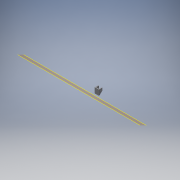
# Autodesk Inventor part: Y belt mount point
Saved by Autodesk Inventor 2016 (Build 200138000, 138)
## iProperties
Created: 2016-05-31
Part Number: Y belt mount point
Material: Generic
Document SubType Name: Modeling
Designer: Scott
Density: 1 g/cm^3
Appearance: Default
Author: Scott
Autodesk Inventor part; units mm, degrees
ref_plane "YZ Plane" through (0, 0, 0) normal (1, 0, 0) x (0, 1, 0)
ref_plane "XZ Plane" through (0, 0, 0) normal (0, 1, 0) x (-1, 0, 0)
ref_plane "XY Plane" through (0, 0, 0) normal (0, 0, 1) x (1, 0, 0)
ref_plane "Work Plane1" through (39.6605, 279.3484, 58.7085) normal (0, 1, 0) x (1, 0, 0)
sketch "Sketch1" plane through (39.6605, 279.3484, 58.7085) normal (0, 1, 0) x (1, 0, 0)
  line L0 (-19.6605, 58.7085) -> (-19.6605, 78.7085) projected
  line L1 (-19.6605, 58.7085) -> (-19.6605, 58.7085) projected
  line L2 (-19.6605, 58.7085) -> (-19.6605, 78.7085) projected
  line L3 (-19.6605, 78.7085) -> (-19.6605, 78.7085) projected
  line L4 (-39.6605, 78.7085) -> (-39.6605, 58.7085) projected
  line L5 (-39.6605, 78.7085) -> (-39.6605, 78.7085) projected
  line L6 (-39.6605, 78.7085) -> (-39.6605, 58.7085) projected
  line L7 (-39.6605, 58.7085) -> (-39.6605, 58.7085) projected
  line L8 (-19.6605, 58.7085) -> (-39.6605, 58.7085)
  line L9 (-39.6605, 58.7085) -> (-39.6605, 53.6285)
  line L10 (-39.6605, 53.6285) -> (-19.6605, 53.6285)
  line L11 (-19.6605, 53.6285) -> (-19.6605, 58.7085)
  dimension "d0" = 5.08
  constraints: 8 end point, 2 parallel, 1 horizontal, 1 perpendicular
  measures "d0" distance of L9.end L8.end
extrude "Extrusion1" add sketch "Sketch1" along normal mid plane 38.1
sketch "Sketch2" plane through (0, 298.3984, 5.08) normal (0, 0, 1) x (1, 0, 0)
  line L0 (20, -38.1) -> (20, 0) projected
  line L1 (0, 0) -> (20, 0) projected
  line L2 (0, -38.1) -> (0, 0) projected
  line L3 (20, -38.1) -> (0, -38.1) projected
  circle A0 centre (10, -7.62) radius 2.5
  point P0 (0, -298.3984)
  dimension "d3" = 5
  dimension "d6" = 7.62
  constraints: 1 centre point
  measures "d3" diameter of A0
  measures "d6" distance from line of L1 A0.centre
extrude "Extrusion3" cut sketch "Sketch2" against normal blind 38.1 contours A0
sketch "Sketch3" plane through (0, 260.2984, 5.08) normal (-1, 0, 0) x (0, 0, 1)
  line L0 (-25.08, 298.5016) -> (-5.08, 298.5016) projected
  line L1 (-25.08, -260.2984) -> (-25.08, 298.5016) projected
  line L2 (-25.08, -260.2984) -> (-5.08, -260.2984) projected
  line L3 (-5.08, -260.2984) -> (-5.08, 298.5016) projected
  line L4 (0, 0) -> (0, 38.1) projected
  line L5 (-5.08, 38.1) -> (0, 38.1) projected
  line L6 (-5.08, 0) -> (-5.08, 38.1) projected
  line L7 (0, 0) -> (-5.08, 0) projected
  line L8 (0, 38.1) -> (-25.08, 38.1)
  line L9 (-25.08, 38.1) -> (-25.08, 18.1)
  line L10 (-25.08, 18.1) -> (0, 18.1)
  line L11 (0, 18.1) -> (0, 38.1)
  dimension "d11" = 20
  constraints: 8 end point, 2 parallel, 1 horizontal, 1 perpendicular, 1 point on line
  measures "d11" distance of L9.end L8.end
extrude "Extrusion4" add sketch "Sketch3" along normal blind 5.08 contours L8 L3 L10 L1 | L5 L4 L10 L3
sketch "Sketch4" plane through (20, 260.2984, 0) normal (1, 0, 0) x (0, 0, -1)
  line L0 (20, 18.1) -> (-5.08, 18.1) projected
  line L1 (-5.08, 18.1) -> (-5.08, 38.1) projected
  line L2 (-5.08, 38.1) -> (20, 38.1) projected
  line L3 (20, 38.1) -> (20, 18.1) projected
  line L4 (-5.08, 18.1) -> (0, 18.1) projected
  line L5 (0, 0) -> (0, 18.1) projected
  line L6 (-5.08, 0) -> (0, 0) projected
  line L7 (-5.08, 0) -> (-5.08, 18.1) projected
  point P0 (0, -260.2984)
extrude "Extrusion5" add sketch "Sketch4" along normal blind 5.08
sketch "Sketch5" plane through (0, 260.2984, 0) normal (-1, 0, 0) x (0, 0, 1)
  line L0 (5.08, 18.1) -> (0, 18.1) projected
  line L1 (0, 0) -> (0, 18.1) projected
  line L2 (5.08, 0) -> (0, 0) projected
  line L3 (5.08, 0) -> (5.08, 18.1) projected
  point P0 (0, -260.2984)
extrude "Extrusion6" add sketch "Sketch5" along normal blind 5.08
sketch "Sketch6" plane through (-5.08, 260.2984, 5.08) normal (-1, 0, 0) x (0, 0, 1)
  line L0 (-25.08, 18.1) -> (-5.08, 18.1) projected
  line L1 (-5.08, 18.1) -> (-5.08, 0) projected
  line L2 (-5.08, 0) -> (0, 0) projected
  line L3 (0, 0) -> (0, 38.1) projected
  line L4 (0, 38.1) -> (-25.08, 38.1) projected
  line L5 (-25.08, 38.1) -> (-25.08, 18.1) projected
  circle A0 centre (-15.08, 28.1) radius 2.5
  point P0 (-5.08, -260.2984)
  dimension "d18" = 5
  constraints: 1 centre point
  measures "d18" diameter of A0
extrude "Extrusion7" cut sketch "Sketch6" along normal mid plane 2540 contours A0
chamfer "Chamfer1" distance 17.4625 angle 45 2 edges at (-2.54, 278.3984, 0) (22.54, 278.3984, 0)
body "Solid1"
